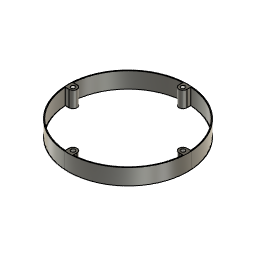
conector fatiado 102 mm v2 (Autodesk Fusion 360 design; units mm, degrees)
Autodesk Fusion 360 part; units mm, degrees
sketch "Esboço2" plane through (0, 0, 0) normal (0, 0, 1) x (1, 0, 0)
  circle A0 centre (0, 0) radius 37.5
  circle A1 centre (0, 0) radius 37
  dimension "d6" = 75
  dimension "d7" = 74
  constraint coincident A0.centre A1.centre
  measures "d6" diameter of A0
  measures "d7" diameter of A1
extrude "Extrusão2" add sketch "Esboço2" along normal blind 190
ref_plane "Plano de trabalho9" through (0, 0, 187) normal (0, 0, 1) x (1, 0, 0)
sketch "Esboço10" plane through (0, 0, 187) normal (0, 0, 1) x (1, 0, 0)
  circle A0 centre (0, 0) radius 34.5 construction
  line L0 (0, 0) -> (-68.1762, 0) construction
  line L1 (0, 0) -> (60, 0) construction
  line L2 (0, 0) -> (0, 45) construction
  line L3 (0, 0) -> (0, -43.1659) construction
  circle A1 centre (34.5, 0) radius 1.5
  line L4 (3, -43) -> (3, -42)
  circle A2 centre (0, 34.5) radius 1.5
  circle A3 centre (-34.5, 0) radius 1.5
  circle A4 centre (0, -34.5) radius 1.5
  arc A5 (34.5, 2.5) -> (34.5, -2.5) centre (34.5, 0) ccw
  arc A6 (-2.5, 34.5) -> (2.5, 34.5) centre (0, 34.5) ccw
  arc A7 (-34.5, -2.5) -> (-34.5, 2.5) centre (-34.5, 0) ccw
  arc A8 (2.5, -34.5) -> (-2.5, -34.5) centre (0, -34.5) ccw
  circle A9 centre (0, 0) radius 37
  line L5 (-36.9154, 2.5) -> (-34.4093, 2.5)
  line L6 (-36.9154, -2.5) -> (-34.4093, -2.5)
  line L7 (34.5, 2.5) -> (36.9154, 2.5)
  line L8 (34.5, -2.5) -> (36.9154, -2.5)
  line L9 (2.5, 36.9154) -> (2.5, 34.4093)
  line L10 (-2.5, 36.9154) -> (-2.5, 34.4093)
  line L11 (-2.5, -34.4093) -> (-2.5, -36.9154)
  line L12 (2.5, -34.4093) -> (2.5, -36.9154)
  dimension "d82" = 69
  dimension "d83" = 3
  dimension "d84" = 2.5
  dimension "d85" = 2.5
  dimension "d87" = 360
  dimension "d89" = 360
  dimension "d90" = 2.5
  constraint coincident A0.centre L0.start
  constraint horizontal L0
  constraint parallel L0 L1
  constraint perpendicular L1 L2
  constraint perpendicular L0 L3
  constraint coincident L1 A1.centre
  constraint coincident A0 A1.centre
  constraint perpendicular L2 L5
  constraint symmetric L1 L5.start L6.start
  constraint symmetric L1 L7.end L8.end
  constraint perpendicular L4 L5
  constraint perpendicular L6 L9
  constraint symmetric L2 L9.start L10.start
  constraint symmetric L2 L12.end L11.end
  constraint concentric A1 A5
  constraint tangent A5 L6
  constraint coincident A5.end L6
  constraint coincident L7.end A9
  constraint coincident L9.start A9
  constraint coincident L5.start A9
  constraint coincident L11.end A9
  constraint coincident A0 L5.end
  constraint coincident A0 L6.end
  constraint coincident A0 L9.end
  constraint coincident A0 L10.end
  constraint coincident A0 L11.start
  constraint coincident A0 L12.start
  constraint tangent A5 L8
  measures "d82" diameter of A0
  measures "d83" diameter of A1
  measures "d84" distance of L1 L5
  measures "d85" distance of L3 L9
  measures "d90" distance of A1.centre L7
extrude "Extrusão12" add sketch "Esboço10" against normal blind 184 contours A5 A9 L7 L8 | A6 A9 L9 L10 | A8 A9 L11 L12 | A7 A9 L5 L6
thread "Rosca3" "ISO Metric profile 3.0 M3x0.5 6H" major diameter 3.086 minor diameter 2.529 pitch 0.5 angle 60 resizes the face on face at (34.5604, -1.4988, 64.3333) on face at (1.4951, -34.6207, 64.3333) on face at (1.4951, 34.3793, 64.3333) on face at (-34.4396, -1.4988, 64.3333)
ref_plane "Plano de trabalho3" through (0, 0, 32) normal (0, 0, 1) x (1, 0, 0)
sketch "Esboço3" plane through (0, 0, 32) normal (0, 0, 1) x (1, 0, 0)
  line L0 (0, 0) -> (0, 37) construction
  line L1 (34.2491, 14) -> (-34.2491, 14)
  circle A0 centre (0, 0) radius 37
  line L2 (31.1288, 20) -> (-31.1288, 20)
  line L3 (32.8634, 17) -> (-32.8634, 17)
  circle A1 centre (0, 0) radius 50
  circle A2 centre (0, 0) radius 37.5
  line L4 (-8, 0) -> (8, 0)
  line L5 (8, 0) -> (8, 36.1248)
  line L6 (-8, 0) -> (-8, 36.1248)
  circle A3 centre (0, 34.5) radius 1.5
  line L7 (1.5, 32.5) -> (1.5, 0)
  arc A4 (-2.5, 34.5) -> (2.5, 34.5) centre (0, 34.5) ccw
  line L8 (-1.5, 32.5) -> (-1.5, 0)
  line L9 (27.8634, 24.3441) -> (27.8634, 11)
  line L10 (27.8634, 11) -> (35.327, 11)
  line L11 (-27.8634, 11) -> (-35.327, 11)
  line L12 (-27.8634, 24.3441) -> (-27.8634, 11)
  line L13 (-30.4631, 21) -> (30.4631, 21)
  line L14 (-34.641, 13) -> (34.641, 13)
  line L15 (0, 32) -> (8, 32)
  line L16 (0, 32) -> (-8, 32)
  dimension "d12" = 6
  dimension "d15" = 3
  dimension "d17" = 75
  dimension "d18" = 100
  dimension "d41" = 14
  dimension "d51" = 8
  dimension "d52" = 16
  dimension "d99" = 3
  dimension "d100" = 2.5
  dimension "d115" = 6.5
  dimension "d123" = 5
  dimension "d124" = 6
  dimension "d143" = 4
  dimension "d144" = 4
  constraint coincident L0.start A0.centre
  constraint vertical L0
  constraint perpendicular L0 L1
  constraint perpendicular L0 L2
  constraint coincident A0 L1.end
  constraint coincident A0 L2.end
  constraint coincident A0 L2.start
  constraint coincident L1.start A0
  constraint perpendicular L0 L3
  constraint concentric A0 A1
  constraint concentric A0 A2
  constraint perpendicular L0 L4
  constraint coincident A0 L5.end
  constraint perpendicular L4 L5
  constraint coincident A0 L6.end
  constraint perpendicular L4 L6
  constraint coincident L0.end A0
  constraint coincident L0 A3.centre
  constraint coincident L0.start L4
  constraint vertical L7
  constraint coincident L7.start A4
  constraint coincident L4 L7.end
  constraint symmetric L0 L7.start L8.start
  constraint symmetric L0 L7.end L8.end
  constraint perpendicular L1 L9
  constraint coincident A0 L9.start
  constraint perpendicular L9 L10
  constraint coincident A0 L10.end
  constraint coincident A0 L3.start
  constraint symmetric L0 L9.start L12.start
  constraint symmetric L0 L9.end L11.start
  constraint symmetric L0 L10.end L11.end
  constraint coincident A0 L3.end
  constraint perpendicular L7 L13
  constraint coincident A0 L13.end
  constraint coincident A0 L13.start
  constraint perpendicular L5 L14
  constraint coincident A0 L14.start
  constraint coincident A0 L14.end
  constraint midpoint A4 L15.start
  constraint coincident L5 L15.end
  constraint tangent A4 L15
  constraint perpendicular L5 L15
  constraint symmetric L0 L15.start L16.start
  constraint symmetric L0 L15.end L16.end
  measures "d12" distance of L1 L2
  measures "d15" distance of L1 L3
  measures "d17" diameter of A2
  measures "d18" diameter of A1
  measures "d41" distance of L1 L0.start
  measures "d51" distance of L0 L5
  measures "d52" distance of L4.start L4.end
  measures "d99" diameter of A3
  measures "d100" distance of L0.end A3.centre
  measures "d115" distance of L5 L7
  measures "d123" distance of L3.start L9
  measures "d124" distance of L3.start L10
  measures "d143" distance of L3 L13
  measures "d144" distance of L3 L14
extrude "Extrusão21" add sketch "Esboço3" along normal blind 6 and the other way blind 6 contours L1 A0 L9 L14 | L1 A0 L3 L9 | A0 L9 L10 L14 | A0 L2 L3 L9 | A0 L2 L9 L13 | A0 L9 L13 | A0 L11 L12 L14 | L1 A0 L12 L14 | L1 A0 L3 L12 | A0 L2 L3 L12 | A0 L12 L13 | A0 L2 L12 L13
sketch "Esboço18" plane through (-27.8634, 0, 0) normal (1, 0, 0) x (0, 1, 0)
  line L0 (24.3441, 26) -> (24.3441, 38)
  line L1 (24.3441, 38) -> (11, 38)
  line L2 (11, 38) -> (11, 26)
  line L3 (11, 26) -> (24.3441, 26)
  circle A0 centre (17, 32) radius 4
  point P0 (11, 32)
  dimension "d166" = 8
  dimension "d167" = 6
  dimension "d168" = 6
  measures "d166" diameter of A0
  measures "d167" distance of A0.centre P0
  measures "d168" distance of L3 A0.centre
ref_plane "Plano de trabalho11" through (0, 0, 0) normal (1, 0, 0) x (0, 1, 0)
extrude "Extrusão23" cut sketch "Esboço18" against normal blind 15 contours A0
extrude "Extrusão7" add sketch "Esboço3" along normal blind 30 and the other way blind 30 contours L1 L5 L7 L14 | L1 L3 L5 L7 | L4 L5 L7 L14 | L2 L3 L5 L7 | L1 L6 L8 L14 | L1 L3 L6 L8 | L2 L5 L7 L13 | L2 L3 L6 L8 | L4 L6 L8 L14 | L5 L7 L13 L15 | A0 L5 L6 L7 A4 L8 L15 L16 | L2 L6 L8 L13 | L6 L8 L13 L16 | L7 A4 L15 | A4 L8 L16
sketch "Esboço19" plane through (27.8634, 0, 0) normal (-1, 0, 0) x (0, -1, 0)
  line L0 (-11, 26) -> (-11, 38)
  line L1 (-11, 38) -> (-24.3441, 38)
  line L2 (-24.3441, 38) -> (-24.3441, 26)
  line L3 (-24.3441, 26) -> (-11, 26)
extrude "Extrusão24" cut sketch "Esboço18" along normal blind 80 contours A0
sketch "Esboço11" plane through (8, 0, 0) normal (1, 0, 0) x (0, 1, 0)
  line L0 (0, 2) -> (36.1248, 2)
  line L1 (36.1248, 2) -> (36.1248, 62)
  line L2 (36.1248, 62) -> (0, 62)
  line L3 (0, 62) -> (0, 2)
  circle A0 centre (17, 32) radius 3
  circle A1 centre (17, 32) radius 9.5
  circle A2 centre (17, 32) radius 12.5
  line L4 (36.1248, 32) -> (36.1248, -5) construction
  line L5 (0, 32) -> (36.1248, 32)
  line L6 (30.1248, 2) -> (8.3278, 22.9976)
  line L7 (30.1248, 62) -> (8.3278, 41.0024)
  line L8 (30.1248, 2) -> (31.9998, 2)
  line L9 (31.9998, 2) -> (31.9998, 32)
  line L10 (30.1248, 62) -> (31.9998, 62)
  line L11 (31.9998, 62) -> (31.9998, 32)
  circle A3 centre (17, 32) radius 4
  point P0 (14, 32)
  point P1 (20, 32)
  dimension "d106" = 6
  dimension "d107" = 19
  dimension "d109" = 25
  dimension "d110" = 6
  dimension "d147" = 1.875
  constraint concentric A0 A1
  constraint coincident A0 P0
  constraint coincident A0 P1
  constraint concentric A0 A2
  constraint midpoint L1 L4.start
  constraint parallel L1 L4
  constraint coincident L0 L6.start
  constraint coincident A2 L6.end
  constraint tangent A2 L6
  constraint symmetric L5 L6.start L7.start
  constraint symmetric L5 L6.end L7.end
  constraint coincident L0 L8.end
  constraint parallel L0 L8
  constraint coincident L5 L9.end
  constraint perpendicular L5 L9
  constraint symmetric L5 L8.end L10.end
  constraint symmetric L5 L9.end L11.end
  measures "d106" diameter of A0
  measures "d107" diameter of A1
  measures "d109" diameter of A2
  measures "d110" distance of L0.end L6.start
  measures "d147" distance of L6.start L8.end
extrude "Extrusão13" cut sketch "Esboço11" against normal blind 16 contours L0 L3 A2 L5 L6 | L0 A2 L5 L6 L8 L9 | L2 L3 A2 L5 L7 | A1 A2 L5 | A1 A2 L5 | L2 A2 L5 L7 L10 L11 | A1 L5 A3 | A1 L5 A3 | A0 L5 A3 | A0 L5 A3 | A0 L5 | A0 L5
ref_plane "Plano de trabalho4" through (0, 0, 150) normal (0, 0, 1) x (1, 0, 0)
sketch "Esboço4" plane through (0, 0, 150) normal (0, 0, 1) x (1, 0, 0)
  circle A0 centre (0, 0) radius 37
  circle A1 centre (0, 0) radius 50
  circle A2 centre (0, 0) radius 37.5
  line L0 (-20, -31.1288) -> (-20, 31.1288)
  line L1 (-17, -32.8634) -> (-17, 32.8634)
  line L2 (-14, -34.2491) -> (-14, 34.2491)
  line L3 (0, 8) -> (0, -8)
  line L4 (0, 8) -> (-36.1248, 8)
  line L5 (0, -8) -> (-36.1248, -8)
  line L6 (0, 0) -> (-37, 0) construction
  circle A3 centre (-34.5, 0) radius 1.5
  line L7 (0, 1.5) -> (-32.5, 1.5)
  arc A4 (-34.5, -2.5) -> (-34.5, 2.5) centre (-34.5, 0) ccw
  line L8 (0, -1.5) -> (-32.5, -1.5)
  line L9 (-24.3441, -27.8634) -> (-11, -27.8634)
  line L10 (-11, -27.8634) -> (-11, -35.327)
  line L11 (-24.3441, 27.8634) -> (-11, 27.8634)
  line L12 (-11, 27.8634) -> (-11, 35.327)
  line L13 (-13, 34.641) -> (-13, -34.641)
  line L14 (-21, 30.4631) -> (-21, -30.4631)
  line L15 (-32, 0) -> (-32, 8)
  line L16 (-32, 0) -> (-32, -8)
  dimension "d28" = 75
  dimension "d29" = 100
  dimension "d38" = 14
  dimension "d39" = 6
  dimension "d40" = 3
  dimension "d43" = 16
  dimension "d44" = 8
  dimension "d101" = 3
  dimension "d102" = 2.5
  dimension "d116" = 6.5
  dimension "d135" = 6
  dimension "d136" = 5
  dimension "d145" = 4
  dimension "d146" = 4
  constraint concentric A0 A1
  constraint coincident A0.centre A1.centre
  constraint vertical L0
  constraint vertical L1
  constraint vertical L2
  constraint coincident A0 L2.start
  constraint coincident A0 L1.start
  constraint coincident A0 L0.start
  constraint coincident A0 L2.end
  constraint coincident A0 L1.end
  constraint coincident A0 L0.end
  constraint vertical L3
  constraint coincident A0 L4.end
  constraint perpendicular L3 L4
  constraint coincident A0 L5.end
  constraint perpendicular L3 L5
  constraint perpendicular L2 L6
  constraint coincident A0 L6.end
  constraint coincident L6 A3.centre
  constraint coincident L3 L7.start
  constraint perpendicular L0 L7
  constraint coincident L7.end A4
  constraint symmetric L6 L7.start L8.start
  constraint symmetric L6 L7.end L8.end
  constraint coincident A0.centre L3
  constraint perpendicular L2 L9
  constraint coincident A0 L10.end
  constraint perpendicular L9 L10
  constraint coincident A0 L9.start
  constraint symmetric L6 L9.start L11.start
  constraint symmetric L6 L9.end L11.end
  constraint symmetric L6 L10.end L12.end
  constraint perpendicular L8 L13
  constraint coincident A0 L13.end
  constraint coincident A0 L13.start
  constraint perpendicular L11 L14
  constraint coincident A0 L14.start
  constraint coincident A0 L14.end
  constraint midpoint A4 L15.start
  constraint coincident L4 L15.end
  constraint tangent A4 L15
  constraint perpendicular L4 L15
  constraint symmetric L6 L15.start L16.start
  constraint symmetric L6 L15.end L16.end
  measures "d28" diameter of A2
  measures "d29" diameter of A1
  measures "d38" distance of A0.centre L2
  measures "d39" distance of L0 L2
  measures "d40" distance of L1 L2
  measures "d43" distance of L4 L5
  measures "d44" distance of L4 L6
  measures "d101" diameter of A3
  measures "d102" distance of L6.end A3.centre
  measures "d116" distance of L4 L7
  measures "d135" distance of L1 L10
  measures "d136" distance of L1.start L9
  measures "d145" distance of L1 L13
  measures "d146" distance of L1 L14
extrude "Extrusão25" add sketch "Esboço4" along normal blind 6 and the other way blind 6 contours A0 L11 L12 L13 | A0 L9 L10 L13 | A0 L2 L11 L13 | A0 L2 L9 L13 | A0 L1 L2 L11 | A0 L1 L2 L9 | A0 L0 L1 L11 | A0 L0 L1 L9 | A0 L0 L11 L14 | A0 L0 L9 L14 | A0 L11 L14 | A0 L9 L14
sketch "Esboço20" plane through (0, 27.8634, 0) normal (0, -1, 0) x (1, 0, 0)
  line L0 (-11, 144) -> (-11, 156)
  line L1 (-11, 156) -> (-24.3441, 156)
  line L2 (-24.3441, 156) -> (-24.3441, 144)
  line L3 (-24.3441, 144) -> (-11, 144)
  circle A0 centre (-17, 150) radius 4
  dimension "d179" = 8
  dimension "d180" = 6
  dimension "d182" = 6
  measures "d179" diameter of A0
  measures "d180" distance of L3 A0.centre
  measures "d182" distance of L0 A0.centre
extrude "Extrusão26" cut sketch "Esboço20" against normal blind 15 contours A0
sketch "Esboço21" plane through (0, -27.8634, 0) normal (0, 1, 0) x (-1, 0, 0)
  line L0 (24.3441, 144) -> (24.3441, 156)
  line L1 (24.3441, 156) -> (11, 156)
  line L2 (11, 156) -> (11, 144)
  line L3 (11, 144) -> (24.3441, 144)
  circle A0 centre (17, 150) radius 4
  dimension "d185" = 8
  dimension "d186" = 6
  dimension "d187" = 6
  measures "d185" diameter of A0
  measures "d186" distance of L2 A0.centre
  measures "d187" distance of L3 A0.centre
extrude "Extrusão27" cut sketch "Esboço21" against normal blind 15 contours A0
extrude "Extrusão6" add sketch "Esboço4" along normal blind 30 and the other way blind 30 contours L2 L4 L7 L13 | L3 L4 L7 L13 | L3 L5 L8 L13 | L2 L5 L8 L13 | L1 L2 L4 L7 | L1 L2 L5 L8 | L0 L1 L4 L7 | L0 L1 L5 L8 | L0 L4 L7 L14 | L0 L5 L8 L14 | A0 L4 L5 L7 A4 L8 L15 L16 | L4 L7 L14 L15 | L5 L8 L14 L16 | L7 A4 L15 | A4 L8 L16
sketch "Esboço13" plane through (0, -8, 0) normal (0, -1, 0) x (1, 0, 0)
  line L0 (0, 120) -> (0, 180)
  line L1 (0, 180) -> (-36.1248, 180)
  line L2 (-36.1248, 180) -> (-36.1248, 120)
  line L3 (-36.1248, 120) -> (0, 120)
  circle A0 centre (-17, 150) radius 3
  circle A1 centre (-17, 150) radius 9.5
  circle A2 centre (-17, 150) radius 12.5
  line L4 (-36.1248, 150) -> (-36.1248, 198.4836) construction
  line L5 (-30.1248, 180) -> (-6.6704, 157.4058)
  line L6 (0, 150) -> (-36.1248, 150)
  line L7 (-30.1248, 120) -> (-6.6704, 142.5942)
  line L8 (-30.1248, 180) -> (-31.9998, 180)
  line L9 (-31.9998, 180) -> (-31.9998, 150)
  line L10 (-30.1248, 120) -> (-31.9998, 120)
  line L11 (-31.9998, 120) -> (-31.9998, 150)
  point P0 (-14, 150)
  point P1 (-20, 150)
  dimension "d117" = 6
  dimension "d118" = 19
  dimension "d119" = 25
  dimension "d120" = 6
  dimension "d148" = 1.875
  constraint coincident A0 P0
  constraint coincident A0 P1
  constraint concentric A0 A1
  constraint concentric A1 A2
  constraint midpoint L2 L4.start
  constraint perpendicular L1 L4
  constraint tangent A2 L5
  constraint coincident L1 L5.start
  constraint symmetric L5.start L6 L7.start
  constraint symmetric L5.end L6 L7.end
  constraint coincident L1 L8.end
  constraint parallel L1 L8
  constraint coincident L6 L9.end
  constraint perpendicular L6 L9
  constraint symmetric L6 L8.end L10.end
  constraint symmetric L6 L9.end L11.end
  measures "d117" diameter of A0
  measures "d118" diameter of A1
  measures "d119" diameter of A2
  measures "d120" distance of L4 L5.start
  measures "d148" distance of L5.start L8.end
extrude "Extrusão14" cut sketch "Esboço13" against normal blind 16 contours L0 L3 A2 L6 L7 | L0 L1 A2 L5 L6 | L3 A2 L6 L7 L10 L11 | A1 A2 L6 | A1 A2 L6 | L1 A2 L5 L6 L8 L9 | A0 A1 L6 | A0 A1 L6 | A0 L6 | A0 L6
ref_plane "Plano de trabalho5" through (0, 0, 0) normal (1, 0, 0) x (0, 1, 0)
ref_plane "Plano de trabalho6" through (0, 0, 0) normal (0, 1, 0) x (0, 0, 1)
ref_plane "Plano de trabalho7" through (0, 0, 134.3) normal (0, 0, 1) x (1, 0, 0)
sketch "Esboço8" plane through (0, 0, 134.3) normal (0, 0, 1) x (1, 0, 0)
  line L0 (46.3444, 0) -> (0, 0) construction
  line L1 (8, 36.1248) -> (8, -36.1248)
  line L2 (-8, -36.1248) -> (-8, 36.1248)
  circle A0 centre (0, 0) radius 37
  line L3 (0, 0) -> (0, 37) construction
  circle A1 centre (0, 34.5) radius 1.5
  circle A2 centre (0, -34.5) radius 1.5
  dimension "d72" = 8
  dimension "d73" = 8
  dimension "d95" = 2.5
  dimension "d96" = 3
  constraint coincident L0.end A0.centre
  constraint horizontal L0
  constraint perpendicular L0 L1
  constraint vertical L2
  constraint coincident L2.end A0
  constraint coincident L2.start A0
  constraint coincident L1.start A0
  constraint coincident L1.end A0
  constraint perpendicular L0 L3
  constraint coincident L3 A1.centre
  constraint coincident A0 L3.end
  constraint symmetric L0 A1 A2
  measures "d72" distance of L1 L3
  measures "d73" distance of L2 L3
  measures "d95" distance of L3.end A1.centre
  measures "d96" diameter of A1
extrude "Extrusão10" add sketch "Esboço8" along normal blind 2 contours L1 L2 A0
ref_plane "Plano de trabalho8" through (0, 0, 45.7) normal (0, 0, 1) x (1, 0, 0)
sketch "Esboço9" plane through (0, 0, 45.7) normal (0, 0, 1) x (1, 0, 0)
  line L0 (0, 0) -> (-37, 0) construction
  line L1 (-36.1248, 8) -> (36.1248, 8)
  line L2 (-36.1248, -8) -> (36.1248, -8)
  circle A0 centre (0, 0) radius 37
  circle A1 centre (-34.5, 0) radius 1.5
  line L3 (0, 0) -> (0, 43.2459) construction
  circle A2 centre (34.5, 0) radius 1.5
  dimension "d77" = 8
  dimension "d78" = 8
  dimension "d97" = 3
  dimension "d98" = 2.5
  constraint coincident L0.start A0.centre
  constraint horizontal L0
  constraint horizontal L1
  constraint horizontal L2
  constraint coincident L1.start A0
  constraint coincident L1.end A0
  constraint coincident L2.end A0
  constraint coincident L2.start A0
  constraint coincident L0.end A0
  constraint coincident L0 A1.centre
  constraint perpendicular L1 L3
  constraint symmetric A1 L3 A2
  measures "d77" distance of L0 L1
  measures "d78" distance of L0 L2
  measures "d97" diameter of A1
  measures "d98" distance of L0.end A1.centre
extrude "Extrusão11" add sketch "Esboço9" along normal blind 2 contours L1 L2 A0
ref_plane "Plano de trabalho10" through (8, 18.0624, 32) normal (1, 0, 0) x (0, 1, 0)
sketch "Esboço16" plane through (-31.9998, 0, 0) normal (1, 0, 0) x (0, 1, 0)
  line L0 (1.5, 180) -> (1.5, 120)
  line L1 (1.5, 120) -> (8, 120)
  line L2 (8, 120) -> (8, 180)
  line L3 (8, 180) -> (1.5, 180)
  line L4 (4.75, 180) -> (4.75, 120) construction
  circle A0 centre (4.75, 170) radius 1.5
  circle A1 centre (4.75, 130) radius 1.5
  line L5 (8, 150) -> (-12.335, 150) construction
  line L6 (0, 2.5) -> (0, 20)
  circle A2 centre (-4.75, 170) radius 1.5
  circle A3 centre (-4.75, 130) radius 1.5
  dimension "d149" = 3
  dimension "d150" = 3
  dimension "d151" = 40
  dimension "d152" = 20
  constraint midpoint L3 L4.start
  constraint midpoint L1 L4.end
  constraint coincident L4 A0.centre
  constraint coincident L4 A1.centre
  constraint midpoint L2 L5.start
  constraint perpendicular L0 L5
  constraint symmetric A0 L6 A2
  constraint symmetric A1 L6 A3
  measures "d149" diameter of A0
  measures "d150" diameter of A1
  measures "d151" distance of A0.centre A1.centre
  measures "d152" distance of A0.centre L5
extrude "Extrusão19" cut sketch "Esboço16" against normal blind 10 contours A0 | A1 | A2 | A3
sketch "Esboço17" plane through (0, 31.9998, 0) normal (0, -1, 0) x (1, 0, 0)
  line L0 (1.5, 62) -> (1.5, 2)
  line L1 (1.5, 2) -> (8, 2)
  line L2 (8, 2) -> (8, 62)
  line L3 (8, 62) -> (1.5, 62)
  line L4 (4.75, 2) -> (4.75, 62) construction
  line L5 (8, 32) -> (-12, 32) construction
  circle A0 centre (4.75, 52) radius 1.5
  circle A1 centre (4.75, 12) radius 1.5
  line L6 (0, 1.75) -> (0, 22.5)
  circle A2 centre (-4.75, 12) radius 1.5
  circle A3 centre (-4.75, 52) radius 1.5
  dimension "d155" = 3
  dimension "d156" = 3
  dimension "d157" = 40
  dimension "d158" = 20
  constraint midpoint L1 L4.start
  constraint midpoint L3 L4.end
  constraint midpoint L2 L5.start
  constraint perpendicular L0 L5
  constraint coincident L4 A0.centre
  constraint coincident L4 A1.centre
  constraint symmetric A0 L6 A3
  constraint symmetric A1 L6 A2
  measures "d155" diameter of A1
  measures "d156" diameter of A0
  measures "d157" distance of A0.centre A1.centre
  measures "d158" distance of L5 A1.centre
extrude "Extrusão20" cut sketch "Esboço17" against normal blind 10 contours A0 | A1 | A2 | A3
thread "Rosca4" "ISO Metric profile 3.0 M3x0.5 6H" major diameter 3.086 minor diameter 2.529 pitch 0.5 angle 60 resizes the face on face at (3.2548, 33.786, 52.1197) on face at (-3.2536, 33.7861, 51.8959) on face at (-3.2536, 33.7861, 11.8959) on face at (3.2548, 33.786, 12.1197)
thread "Rosca5" "ISO Metric profile 3.0 M3x0.5 6H" major diameter 3.086 minor diameter 2.529 pitch 0.5 angle 60 resizes the face on face at (-33.786, 3.2548, 130.1197) on face at (-33.7861, -3.2536, 169.8959) on face at (-33.786, 3.2548, 170.1197) on face at (-33.7861, -3.2536, 129.8959)
sketch "Esboço22" plane through (0, 0, 136.3) normal (0, 0, 1) x (-1, 0, 0)
  line L0 (2.5, 36.9154) -> (2.5, 34.5)
  arc A0 (-2.5, 34.5) -> (2.5, 34.5) centre (0, 34.5) ccw
  line L1 (-2.5, 34.5) -> (-2.5, 36.9154)
  arc A1 (-2.5, 36.9154) -> (-8, 36.1248) centre (0, 0) ccw
  line L2 (-8, 36.1248) -> (-8, -36.1248)
  arc A2 (-8, -36.1248) -> (-2.5, -36.9154) centre (0, 0) ccw
  line L3 (-2.5, -36.9154) -> (-2.5, -34.5)
  arc A3 (2.5, -34.5) -> (-2.5, -34.5) centre (0, -34.5) ccw
  line L4 (2.5, -34.5) -> (2.5, -36.9154)
  arc A4 (2.5, -36.9154) -> (8, -36.1248) centre (0, 0) ccw
  line L5 (8, -36.1248) -> (8, 36.1248)
  arc A5 (8, 36.1248) -> (2.5, 36.9154) centre (0, 0) ccw
  line L6 (0, 0) -> (-21, 0) construction
  line L7 (0, 0) -> (0, -19.3) construction
  line L8 (2, -15.8) -> (-2, -15.8)
  arc A6 (-2, -15.8) -> (-2, -22.8) centre (-2, -19.3) ccw
  line L9 (-2, -22.8) -> (2, -22.8)
  arc A7 (2, -22.8) -> (2, -15.8) centre (2, -19.3) ccw
  line L10 (2, -19.3) -> (-2, -19.3) construction
  arc A8 (-2, 22.8) -> (-2, 15.8) centre (-2, 19.3) ccw
  line L11 (2, 15.8) -> (-2, 15.8)
  arc A9 (2, 15.8) -> (2, 22.8) centre (2, 19.3) ccw
  line L12 (-2, 22.8) -> (2, 22.8)
  circle A10 centre (0, 10.8) radius 1.5 construction
  line L13 (2, 19.3) -> (-2, 19.3) construction
  line L14 (2, 12.3) -> (-2, 12.3)
  arc A11 (-2, 12.3) -> (-2, 9.3) centre (-2, 10.8) ccw
  line L15 (-2, 9.3) -> (2, 9.3)
  arc A12 (2, 9.3) -> (2, 12.3) centre (2, 10.8) ccw
  line L16 (2, 10.8) -> (-2, 10.8) construction
  line L17 (2, 26.3) -> (-2, 26.3)
  arc A13 (2, 26.3) -> (2, 29.3) centre (2, 27.8) ccw
  line L18 (-2, 29.3) -> (2, 29.3)
  arc A14 (-2, 29.3) -> (-2, 26.3) centre (-2, 27.8) ccw
  arc A15 (2, -29.3) -> (2, -26.3) centre (2, -27.8) ccw
  line L19 (2, -26.3) -> (-2, -26.3)
  arc A16 (-2, -26.3) -> (-2, -29.3) centre (-2, -27.8) ccw
  line L20 (-2, -29.3) -> (2, -29.3)
  arc A17 (2, -12.3) -> (2, -9.3) centre (2, -10.8) ccw
  line L21 (-2, -9.3) -> (2, -9.3)
  arc A18 (-2, -9.3) -> (-2, -12.3) centre (-2, -10.8) ccw
  line L22 (2, -12.3) -> (-2, -12.3)
  point P0 (0, -19.3)
  point P1 (0, 10.8)
  dimension "d191" = 19.3
  dimension "d195" = 2
  dimension "d196" = 3.5
  dimension "d204" = 3
  dimension "d205" = 8.5
  dimension "d230" = 1.5
  dimension "d231" = 4
  constraint coincident A1.centre A2.centre
  constraint horizontal L6
  constraint perpendicular L6 L7
  constraint tangent L8 A6
  constraint tangent A6 L9
  constraint parallel L8 L9
  constraint tangent L9 A7
  constraint tangent L8 A7
  constraint perpendicular L7 L10
  constraint coincident P0 L7.end
  constraint midpoint L10 P0
  constraint symmetric L6 L8.start L11.start
  constraint symmetric L6 L8.end A8.end
  constraint symmetric L6 A6.end A8.start
  constraint symmetric L6 L9.end A9.end
  constraint symmetric L6 A6 A8
  constraint symmetric L6 A7 A9
  constraint vertical A1.centre P1
  constraint coincident A9.centre L13.start
  constraint coincident A8.centre L13.end
  constraint tangent L14 A11
  constraint tangent A11 L15
  constraint parallel L14 L15
  constraint tangent L15 A12
  constraint tangent L14 A12
  constraint horizontal L16
  constraint coincident P1 A10.centre
  constraint midpoint L16 P1
  constraint symmetric L13 L14.start L17.start
  constraint symmetric L13 L14.end L17.end
  constraint symmetric L13 A11.end L18.start
  constraint symmetric L13 L15.end A13.end
  constraint symmetric L13 A11 A14
  constraint symmetric L13 A12 A13
  constraint symmetric L6 L14.start A17.start
  constraint symmetric L6 L14.end A18.end
  constraint symmetric L6 A11.end L21.start
  constraint symmetric L6 L15.end A17.end
  constraint symmetric L6 A11 A18
  constraint symmetric L6 A12 A17
  constraint symmetric L6 L17.start A15.end
  constraint symmetric L6 L17.end L19.end
  constraint symmetric L6 A13.end A15.start
  constraint symmetric L6 A13 A15
  constraint symmetric L6 L18.start A16.end
  constraint symmetric L6 A14 A16
  measures "d191" distance of A1.centre P0
  measures "d195" distance of A6.centre P0
  measures "d196" radius of A7
  measures "d204" diameter of A10
  measures "d205" vertical distance of A9.centre P1
  measures "d230" radius of A11
  measures "d231" distance of A11.end L15.end
extrude "Extrusão28" cut sketch "Esboço22" against normal blind 5 contours L8 A6 L9 A7 | A8 L11 A9 L12 | L14 A11 L15 A12 | L17 A13 L18 A14 | A15 L19 A16 L20 | A17 L21 A18 L22
sketch "Esboço23" plane through (0, 0, 45.7) normal (0, 0, -1) x (1, 0, 0)
  line L0 (36.9154, -2.5) -> (34.5, -2.5)
  arc A0 (34.5, 2.5) -> (34.5, -2.5) centre (34.5, 0) ccw
  line L1 (34.5, 2.5) -> (36.9154, 2.5)
  arc A1 (36.9154, 2.5) -> (36.1248, 8) centre (0, 0) ccw
  line L2 (36.1248, 8) -> (-36.1248, 8)
  arc A2 (-36.1248, 8) -> (-36.9154, 2.5) centre (0, 0) ccw
  line L3 (-36.9154, 2.5) -> (-34.5, 2.5)
  arc A3 (-34.5, -2.5) -> (-34.5, 2.5) centre (-34.5, 0) ccw
  line L4 (-34.5, -2.5) -> (-36.9154, -2.5)
  arc A4 (-36.9154, -2.5) -> (-36.1248, -8) centre (0, 0) ccw
  line L5 (-36.1248, -8) -> (36.1248, -8)
  arc A5 (36.1248, -8) -> (36.9154, -2.5) centre (0, 0) ccw
  line L6 (0, 0) -> (0, -19) construction
  line L7 (0, 0) -> (19.3, 0)
  line L8 (15.8, 2.5) -> (15.8, -2.5)
  arc A6 (15.8, -2.5) -> (22.8, -2.5) centre (19.3, -2.5) ccw
  line L9 (22.8, -2.5) -> (22.8, 2.5)
  arc A7 (22.8, 2.5) -> (15.8, 2.5) centre (19.3, 2.5) ccw
  line L10 (19.3, 2.5) -> (19.3, -2.5) construction
  line L11 (-15.8, 2.5) -> (-15.8, -2.5)
  arc A8 (-15.8, 2.5) -> (-22.8, 2.5) centre (-19.3, 2.5) ccw
  line L12 (-22.8, -2.5) -> (-22.8, 2.5)
  arc A9 (-22.8, -2.5) -> (-15.8, -2.5) centre (-19.3, -2.5) ccw
  circle A10 centre (10.8, 0) radius 1.5 construction
  circle A11 centre (27.8, 0) radius 1.5 construction
  line L13 (9.3, 2.5) -> (9.3, -2.5)
  arc A12 (9.3, -2.5) -> (12.3, -2.5) centre (10.8, -2.5) ccw
  line L14 (12.3, -2.5) -> (12.3, 2.5)
  arc A13 (12.3, 2.5) -> (9.3, 2.5) centre (10.8, 2.5) ccw
  line L15 (10.8, 2.5) -> (10.8, -2.5) construction
  line L16 (26.3, -2.5) -> (26.3, 2.5)
  arc A14 (26.3, -2.5) -> (29.3, -2.5) centre (27.8, -2.5) ccw
  line L17 (29.3, 2.5) -> (29.3, -2.5)
  arc A15 (29.3, 2.5) -> (26.3, 2.5) centre (27.8, 2.5) ccw
  line L18 (-12.3, -2.5) -> (-12.3, 2.5)
  arc A16 (-12.3, -2.5) -> (-9.3, -2.5) centre (-10.8, -2.5) ccw
  line L19 (-9.3, 2.5) -> (-9.3, -2.5)
  arc A17 (-9.3, 2.5) -> (-12.3, 2.5) centre (-10.8, 2.5) ccw
  line L20 (-26.3, -2.5) -> (-26.3, 2.5)
  arc A18 (-29.3, -2.5) -> (-26.3, -2.5) centre (-27.8, -2.5) ccw
  line L21 (-29.3, 2.5) -> (-29.3, -2.5)
  arc A19 (-26.3, 2.5) -> (-29.3, 2.5) centre (-27.8, 2.5) ccw
  point P0 (19.3, 0)
  point P1 (10.8, 0)
  dimension "d199" = 3.5
  dimension "d200" = 5
  dimension "d201" = 19.3
  dimension "d206" = 3
  dimension "d207" = 8.5
  dimension "d228" = 2.5
  dimension "d229" = 1.5
  constraint coincident A1.centre A2.centre
  constraint vertical L6
  constraint perpendicular L6 L7
  constraint tangent L8 A6
  constraint tangent A6 L9
  constraint parallel L8 L9
  constraint tangent L9 A7
  constraint tangent L8 A7
  constraint perpendicular L7 L10
  constraint coincident P0 L7.end
  constraint midpoint L10 P0
  constraint symmetric L6 L8.start L11.start
  constraint symmetric L6 L8.end L11.end
  constraint symmetric L6 A6.end L12.start
  constraint symmetric L6 L9.end A8.end
  constraint symmetric L6 A6 A9
  constraint symmetric L6 A7 A8
  constraint coincident L7 P1
  constraint symmetric L10 A10 A11
  constraint tangent L13 A12
  constraint tangent A12 L14
  constraint parallel L13 L14
  constraint tangent L14 A13
  constraint tangent L13 A13
  constraint perpendicular L7 L15
  constraint coincident P1 A10.centre
  constraint midpoint L15 P1
  constraint symmetric L10 L13.start L17.start
  constraint symmetric L10 L13.end A14.end
  constraint symmetric L10 A12.end L16.start
  constraint symmetric L10 L14.end L16.end
  constraint symmetric L10 A12 A14
  constraint symmetric L10 A13 A15
  constraint symmetric L6 L13.start L19.start
  constraint symmetric L6 L13.end A16.end
  constraint symmetric L6 A12.end L18.start
  constraint symmetric L6 L14.end L18.end
  constraint symmetric L6 A12 A16
  constraint symmetric L6 A13 A17
  constraint symmetric L6 L16.start L20.start
  constraint symmetric L6 L16.end L20.end
  constraint symmetric L6 A14.end A18.start
  constraint symmetric L6 A14 A18
  constraint symmetric L6 L17.start L21.start
  constraint symmetric L6 A15 A19
  measures "d199" radius of A6
  measures "d200" distance of L8.start L8.end
  measures "d201" distance of A1.centre P0
  measures "d206" diameter of A10
  measures "d207" distance of P0 P1
  measures "d228" distance of P1 A12.centre
  measures "d229" radius of A12
extrude "Extrusão29" cut sketch "Esboço23" against normal blind 10 contours L7 L13 L14 A13 | L7 L13 A12 L14 | L8 A6 L9 A7 | L11 A8 L12 A9 | L16 A14 L17 A15 | L20 A18 L21 A19
ref_plane "Plano de trabalho12" through (0, 0, 106.3) normal (0, 0, 1) x (1, 0, 0)
sketch "Esboço24" plane through (0, 0, 106.3) normal (0, 0, 1) x (1, 0, 0)
  line L0 (0, 0) -> (28.1868, 0) construction
  line L1 (16, 0) -> (16, 33.3617)
  circle A0 centre (0, 0) radius 37
  line L2 (16, 0) -> (16, -33.3617)
  line L3 (0, 0) -> (0, 19.3) construction
  line L4 (-16, 0) -> (-16, 33.3617)
  line L5 (-16, 0) -> (-16, -33.3617)
  line L6 (-2, 6.8) -> (2, 6.8)
  arc A1 (2, 6.8) -> (2, 31.8) centre (2, 19.3) ccw
  line L7 (2, 31.8) -> (-2, 31.8)
  arc A2 (-2, 31.8) -> (-2, 6.8) centre (-2, 19.3) ccw
  line L8 (-2, 19.3) -> (2, 19.3) construction
  arc A3 (2, -31.8) -> (2, -6.8) centre (2, -19.3) ccw
  arc A4 (-2, -6.8) -> (-2, -31.8) centre (-2, -19.3) ccw
  line L9 (-2, -6.8) -> (2, -6.8)
  line L10 (2, -31.8) -> (-2, -31.8)
  circle A5 centre (0, 34.5) radius 1.5
  circle A6 centre (0, -34.5) radius 1.5
  point P0 (0, 19.3)
  dimension "d209" = 16
  dimension "d210" = 12.5
  dimension "d211" = 4
  dimension "d212" = 19.3
  dimension "d215" = 3
  dimension "d216" = 34.5
  constraint coincident L0.start A0.centre
  constraint horizontal L0
  constraint coincident L0 L1.start
  constraint perpendicular L0 L1
  constraint coincident L1.end A0
  constraint coincident A0 L2.end
  constraint perpendicular L0 L2
  constraint perpendicular L0 L3
  constraint symmetric L1.start L3 L4.start
  constraint symmetric L1.end L3 L4.end
  constraint symmetric L2.end L3 L5.end
  constraint tangent L6 A1
  constraint tangent A1 L7
  constraint parallel L6 L7
  constraint tangent L7 A2
  constraint tangent L6 A2
  constraint perpendicular L3 L8
  constraint coincident P0 L3.end
  constraint midpoint L8 P0
  constraint symmetric L0 L6.start A4.start
  constraint symmetric L0 L6.end A3.end
  constraint symmetric L0 A1.end A3.start
  constraint symmetric L0 L7.end A4.end
  constraint symmetric L0 A1 A3
  constraint symmetric L0 A2 A4
  constraint symmetric L0 A5 A6
  measures "d209" distance of L0.start L1
  measures "d210" radius of A1
  measures "d211" distance of A2.centre A1.centre
  measures "d212" distance of L0.start L3.end
  measures "d215" diameter of A5
  measures "d216" distance of L0.start A5.centre
ref_plane "Plano de trabalho13" through (0, 0, 55.7) normal (0, 0, -1) x (-1, 0, 0)
ref_plane "Plano de trabalho14" through (0, 0, 60) normal (0, 0, 1) x (1, 0, 0)
sketch "Esboço25" plane through (0, 0, 55.7) normal (0, 0, -1) x (1, 0, 0)
  line L0 (-33.3617, 16) -> (33.3617, 16)
  circle A0 centre (0, 0) radius 37
  line L1 (0, 0) -> (-19.3, 0) construction
  line L2 (-33.3617, -16) -> (33.3617, -16)
  line L3 (-6.8, -2) -> (-6.8, 2)
  arc A1 (-6.8, 2) -> (-31.8, 2) centre (-19.3, 2) ccw
  line L4 (-31.8, 2) -> (-31.8, -2)
  arc A2 (-31.8, -2) -> (-6.8, -2) centre (-19.3, -2) ccw
  line L5 (-19.3, -2) -> (-19.3, 2) construction
  circle A3 centre (-34.5, 0) radius 1.5
  line L6 (0, 0) -> (0, -12) construction
  arc A4 (31.8, 2) -> (6.8, 2) centre (19.3, 2) ccw
  line L7 (6.8, -2) -> (6.8, 2)
  arc A5 (6.8, -2) -> (31.8, -2) centre (19.3, -2) ccw
  circle A6 centre (34.5, 0) radius 1.5
  line L8 (31.8, 2) -> (31.8, -2)
  point P0 (-19.3, 0)
  dimension "d219" = 16
  dimension "d220" = 12.5
  dimension "d221" = 4
  dimension "d222" = 19.3
  dimension "d224" = 34.5
  dimension "d225" = 3
  constraint horizontal L0
  constraint coincident L0.start A0
  constraint coincident L0.end A0
  constraint coincident A0.centre L1.start
  constraint horizontal L1
  constraint symmetric L0.start L1 L2.start
  constraint symmetric L0.end L1 L2.end
  constraint tangent L3 A1
  constraint tangent A1 L4
  constraint parallel L3 L4
  constraint tangent L4 A2
  constraint tangent L3 A2
  constraint perpendicular L1 L5
  constraint coincident P0 L1.end
  constraint midpoint L5 P0
  constraint perpendicular L1 L6
  constraint symmetric L3.start L6 L7.start
  constraint symmetric L3.end L6 A4.end
  constraint symmetric A1.end L6 A4.start
  constraint symmetric L4.end L6 A5.end
  constraint symmetric A1 L6 A4
  constraint symmetric A2 L6 A5
  constraint symmetric A3 L6 A6
  measures "d219" distance of A0.centre L0
  measures "d220" radius of A1
  measures "d221" distance of A2.centre A1.centre
  measures "d222" distance of A0.centre L1.end
  measures "d224" distance of A0.centre A3.centre
  measures "d225" diameter of A3
ref_plane "Plano de trabalho15" through (0, 0, 102) normal (0, 0, 1) x (1, 0, 0)
ref_plane "Plano de trabalho16" through (0, 0, 112) normal (0, 0, 1) x (1, 0, 0)
sketch "Esboço26" plane through (0, 0, 102) normal (0, 0, 1) x (1, 0, 0)
  circle A0 centre (0, 0) radius 42.8513
  constraint coincident A0.centre origin
extrude "Extrusão32" cut sketch "Esboço26" against normal blind 200
sketch "Esboço27" plane through (0, 0, 112) normal (0, 0, 1) x (1, 0, 0)
  circle A0 centre (0, 0) radius 44.9971
  constraint coincident A0.centre origin
extrude "Extrusão33" cut sketch "Esboço27" along normal blind 100
